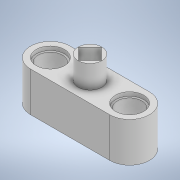
# Autodesk Inventor part: VexLegoCoupler
Saved by Autodesk Inventor 2020 (Build 240168000, 168)
## iProperties
Created: 2020-02-28
Part Number: VexLegoCoupler
Material: Generic
Document SubType Name: Modeling
Designer: Luke
Density: 1 g/cm^3
Appearance: Default
Author: Luke
Autodesk Inventor part; units mm, degrees
ref_plane "YZ Plane" through (0, 0, 0) normal (1, 0, 0) x (0, 1, 0)
ref_plane "XZ Plane" through (0, 0, 0) normal (0, 1, 0) x (-1, 0, 0)
ref_plane "XY Plane" through (0, 0, 0) normal (0, 0, 1) x (1, 0, 0)
sketch "Sketch1" plane through (0, 0, 0) normal (0, 1, 0) x (-1, 0, 0)
  line L0 (-8.001, 0) -> (8.001, 0) construction
  line L1 (-8.001, -4.0005) -> (8.001, -4.0005)
  line L2 (8.001, 4.0005) -> (-8.001, 4.0005)
  arc A0 (-8.001, 4.0005) -> (-8.001, -4.0005) centre (-8.001, 0) ccw
  arc A1 (8.001, -4.0005) -> (8.001, 4.0005) centre (8.001, 0) ccw
  line L3 (-2.3169, 0) -> (0, 2.3169)
  line L4 (0, 2.3169) -> (2.3169, 0)
  line L5 (2.3169, 0) -> (0, -2.3169)
  line L6 (0, -2.3169) -> (-2.3169, 0)
  line L7 (-2.3169, 0) -> (2.3169, 0) construction
  line L8 (0, 2.3169) -> (0, -2.3169) construction
  point P0 (0, 0)
  dimension "d0" = 8.001
  dimension "d1" = 8.001
  dimension "d2" = 3.2766
  dimension "d3" = 3.2766
  constraints: 20 end point, 4 point on circle, 4 tangent, 3 parallel, 2 centre point, 1 horizontal, 1 midpoint, 1 perpendicular
  measures "d0" distance of point (0, 0) L0.end
  measures "d1" diameter of A1
  measures "d2" distance of L4.end L5.end
  measures "d3" distance of L3.end L4.end
extrude "Extrusion1" add sketch "Sketch1" along normal blind 8.001
sketch "Sketch2" plane through (0, 8.001, 0) normal (0, 1, 0) x (1, 0, 0)
  circle A0 centre (-8.001, 0) radius 2.8575
  point P0 (0, 0)
  dimension "d6" = 8.001
  dimension "d7" = 5.715
  constraints: 1 centre point, 1 coincident
  measures "d6" distance of point (0, 0) point (-8.001, 0)
  measures "d7" diameter of A0
extrude "Extrusion2" cut sketch "Sketch2" against normal blind 0.7874
sketch "Sketch3" plane through (0, 8.001, 0) normal (0, 1, 0) x (1, 0, 0)
  circle A0 centre (8.001, 0) radius 2.8575
  point P0 (0, 0)
  dimension "d10" = 8.001
  dimension "d11" = 5.715
  constraints: 1 centre point, 1 coincident
  measures "d10" distance of point (0, 0) point (8.001, 0)
  measures "d11" diameter of A0
extrude "Extrusion3" cut sketch "Sketch3" against normal blind 0.7874
sketch "Sketch4" plane through (0, 0, 0) normal (0, -1, 0) x (1, 0, 0)
  circle A0 centre (8.001, 0) radius 2.8575 projected
  circle A1 centre (8.001, 0) radius 2.8575
  point P0 (0, 0)
  constraints: 1 centre point, 1 coincident
extrude "Extrusion4" cut sketch "Sketch4" against normal blind 0.7874
sketch "Sketch5" plane through (0, 0, 0) normal (0, -1, 0) x (1, 0, 0)
  circle A0 centre (-8.001, 0) radius 2.8575 projected
  circle A1 centre (-8.001, 0) radius 2.8575
  point P0 (0, 0)
  constraints: 1 centre point, 1 coincident
extrude "Extrusion5" cut sketch "Sketch5" against normal blind 0.7874
sketch "Sketch6" plane through (-8.001, 7.2136, 0) normal (0, 1, 0) x (1, 0, 0)
  circle A0 centre (0, 0) radius 2.4511
  point P0 (8.001, 0)
  dimension "d18" = 4.9022
  constraints: 1 centre point
  measures "d18" diameter of A0
extrude "Extrusion6" cut sketch "Sketch6" against normal through all
sketch "Sketch7" plane through (8.001, 7.2136, 0) normal (0, 1, 0) x (1, 0, 0)
  circle A0 centre (0, 0) radius 2.4511
  point P0 (-8.001, 0)
  dimension "d21" = 4.9022
  constraints: 1 centre point
  measures "d21" diameter of A0
extrude "Extrusion7" cut sketch "Sketch7" against normal through all
sketch "Sketch8" plane through (0, 8.001, 0) normal (0, 1, 0) x (1, 0, 0)
  circle A0 centre (0, 0) radius 2.4003
  dimension "d24" = 4.8006
  constraints: 1 centre point, 1 coincident
  measures "d24" diameter of A0
extrude "Extrusion8" add sketch "Sketch8" along normal blind 4.6482
sketch "Sketch9" plane through (0, 12.6492, 0) normal (0, 1, 0) x (1, 0, 0)
  line L0 (2.3169, 0) -> (0, 2.3169)
  line L1 (0, 2.3169) -> (-2.3169, 0)
  line L2 (-2.3169, 0) -> (0, -2.3169)
  line L3 (0, -2.3169) -> (2.3169, 0)
  circle A0 centre (0, 0) radius 2.4003 projected
  line L4 (-1.6383, -1.6383) -> (1.6383, 1.6383) construction
  line L5 (1.6383, -1.6383) -> (-1.6383, 1.6383) construction
  dimension "d27" = 3.2766
  dimension "d28" = 3.2766
  constraints: 12 end point, 2 midpoint, 2 parallel, 1 perpendicular
  measures "d27" distance of L2.end L1.end
  measures "d28" distance of L1.end L0.end
extrude "Extrusion9" cut sketch "Sketch9" against normal blind 4.6482 contours L3 L2 L1 L0
body "Solid1"
